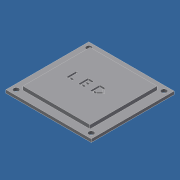
# Autodesk Inventor part: P1704_014_Display
Saved by Autodesk Inventor 2019 (Build 230136000, 136)
## iProperties
Created: 2019-05-23
Part Number: P1704_014_Display
Project: Nom Projet
Material: .
Description: Nom pièce
Document SubType Name: Modeling
Designer: Adel.KAHRIMANOVIC
Authority: brut Ø
Density: 0.001 g/cm^3
Appearance: Par défaut
Author: Adel.KAHRIMANOVIC
Material number: ---
Autodesk Inventor part; units mm, degrees
ref_plane "Plan YZ" through (0, 0, 0) normal (1, 0, 0) x (0, 1, 0)
ref_plane "Plan XZ" through (0, 0, 0) normal (0, 1, 0) x (-1, 0, 0)
ref_plane "Plan XY" through (0, 0, 0) normal (0, 0, 1) x (1, 0, 0)
sketch "Esquisse1" plane through (0, 0, 0) normal (0, 0, 1) x (1, 0, 0)
  line L0 (0, 0) -> (43.25, 0)
  line L1 (43.25, 0) -> (43.25, 42)
  line L2 (43.25, 42) -> (0, 42)
  line L3 (0, 42) -> (0, 0)
  dimension "d0" = 43.25
  dimension "d1" = 42
  constraints: 8 end point, 2 parallel, 1 horizontal, 1 perpendicular
  measures "d0" distance of L0.start L0.end
  measures "d1" distance of L0.end L1.end
extrude "Extrusion1" add sketch "Esquisse1" along normal blind 1.6
sketch "Esquisse6" plane through (0, 0, 1.6) normal (0, 0, 1) x (1, 0, 0)
  line L0 (4.625, 38) -> (38.625, 38)
  line L1 (38.625, 38) -> (38.625, 4)
  line L2 (38.625, 4) -> (4.625, 4)
  line L3 (4.625, 4) -> (4.625, 38)
  line L4 (0, 27.3284) -> (4.625, 27.3284) construction
  line L5 (43.25, 21) -> (38.625, 21) construction
  line L6 (19.4191, 4) -> (19.4191, 0) construction
  line L7 (15.7943, 42) -> (15.7943, 38) construction
  line L8 (0, 0) -> (43.25, 0) construction
  line L9 (43.25, 42) -> (0, 42) construction
  line L10 (43.25, 0) -> (43.25, 42) construction
  line L11 (0, 42) -> (0, 0) construction
  dimension "d4" = 34
  dimension "d5" = 34
  constraints: 16 end point, 6 point on line, 4 parallel, 3 horizontal, 2 midpoint, 2 vertical, 1 perpendicular
  measures "d4" distance of L0.start L0.end
  measures "d5" distance of L0.end L1.end
extrude "Extrusion2" add sketch "Esquisse6" along normal blind 1.9
sketch "Esquisse7" plane through (0, 0, 1.6) normal (0, 0, 1) x (1, 0, 0)
  line L0 (43.25, 0) -> (43.25, 42) projected
  line L1 (43.25, 42) -> (0, 42) projected
  point P0 (0, 0)
  point P1 (40.71, 39.46)
  dimension "d21" = 2.54
  dimension "d22" = 2.54
  measures "d21" distance from line of L0 point (40.71, 39.46)
  measures "d22" distance from line of point (40.71, 39.46) L1
hole "Perçage1" at (40.71, 39.46, 1.6) direction (0, 0, -1) diameter 2.7 end through all
pattern_linear "Réseau rectangulaire1" count 2 spacing 36.9 along (0, -1, 0) count 2 spacing 38.1 along (-1, 0, 0) of "Perçage1"
sketch "Esquisse8" plane through (0, 0, 3.5) normal (0, 0, 1) x (1, 0, 0)
  line L0 (11.625, 24) -> (11.625, 19)
  line L1 (11.625, 19) -> (14.625, 19)
  line L2 (14.625, 19) -> (14.625, 20)
  line L3 (14.625, 20) -> (12.625, 20)
  line L4 (12.625, 20) -> (12.625, 24)
  line L5 (12.625, 24) -> (11.625, 24)
  line L6 (17.625, 24) -> (17.625, 19)
  line L7 (17.625, 19) -> (20.625, 19)
  line L8 (20.625, 19) -> (20.625, 20)
  line L9 (20.625, 20) -> (18.625, 20)
  line L10 (18.625, 20) -> (18.625, 21)
  line L11 (18.625, 21) -> (20.625, 21)
  line L12 (20.625, 21) -> (20.625, 22)
  line L13 (20.625, 22) -> (18.625, 22)
  line L14 (18.625, 22) -> (18.625, 23)
  line L15 (20.625, 23) -> (20.625, 24)
  line L16 (20.625, 24) -> (17.625, 24)
  line L17 (17.625, 24) -> (17.625, 24)
  line L18 (18.625, 23) -> (20.625, 23)
  line L19 (23.625, 19) -> (23.625, 24)
  line L20 (23.625, 24) -> (26.125, 24)
  line L21 (26.125, 24) -> (28.625, 21.5)
  line L22 (28.625, 21.5) -> (26.125, 19)
  line L23 (26.125, 19) -> (23.625, 19)
  line L24 (24.625, 20) -> (24.625, 23)
  line L25 (4.625, 38) -> (4.625, 4) projected
  line L26 (4.625, 4) -> (38.625, 4) projected
  line L27 (24.625, 20) -> (26.125, 20)
  line L28 (26.125, 20) -> (27.625, 21.5)
  line L29 (24.625, 23) -> (26.125, 23)
  line L30 (26.125, 23) -> (27.625, 21.5)
  point P0 (0, 0)
  dimension "d23" = 5
  dimension "d24" = 4
  dimension "d25" = 1
  dimension "d26" = 7
  dimension "d27" = 3
  dimension "d28" = 3
  dimension "d29" = 3
  dimension "d30" = 3
  dimension "d31" = 15
  dimension "d32" = 5
  dimension "d33" = 1
  dimension "d34" = 1
  dimension "d35" = 1
  dimension "d36" = 1
  dimension "d37" = 2
  dimension "d38" = 1
  dimension "d39" = 1
  dimension "d40" = 1
  dimension "d41" = 45
  dimension "d42" = 45
  dimension "d43" = 1
  dimension "d45" = 5
  constraints: 58 end point, 15 point on line, 14 perpendicular, 3 parallel, 2 horizontal, 2 vertical
  measures "d23" distance of L0.start L0.end
  measures "d24" distance between parallel lines of L5 L3
  measures "d25" distance between parallel lines of L0 L4
  measures "d26" distance between parallel lines of L0 L25
  measures "d27" distance of L0.end L1.end
  measures "d28" distance of L6.end L7.end
  measures "d29" distance between parallel lines of L2 L6
  measures "d30" distance between parallel lines of L8 L19
  measures "d31" distance between parallel lines of L26 L1
  measures "d32" distance between parallel lines of L7 L16
  measures "d33" distance of L9.end L10.end
  measures "d34" distance of L11.end L12.end
  measures "d35" distance of L13.end L14.end
  measures "d36" distance between parallel lines of L6 L14
  measures "d37" distance of L14.end L15.start
  measures "d38" distance between parallel lines of L19 L24
  measures "d39" distance between parallel lines of L23 L27
  measures "d40" distance between parallel lines of L20 L29
  measures "d41" angle of L23 L22
  measures "d42" angle of L20 L21
  measures "d43" distance of L21.end L28.end
  measures "d45" distance from line of L19 L21.end
extrude "Extrusion3" cut sketch "Esquisse8" against normal blind 1
